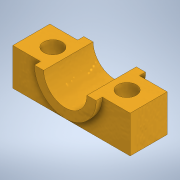
# Autodesk Inventor part: Part22
Saved by Autodesk Inventor 2020 (Build 240168000, 168)
## iProperties
Created: 2021-10-20
Part Number: Part22
Material: Brass, Soft Yellow, Welded
Document SubType Name: Modeling
Designer: simon.erikssonwestl
Density: 8.5 g/cm^3
Appearance: Weld - Brass
Author: simon.erikssonwestl
Autodesk Inventor part; units mm, degrees
ref_plane "YZ Plane" through (0, 0, 0) normal (1, 0, 0) x (0, 1, 0)
ref_plane "XZ Plane" through (0, 0, 0) normal (0, 1, 0) x (-1, 0, 0)
ref_plane "XY Plane" through (0, 0, 0) normal (0, 0, 1) x (1, 0, 0)
sketch "Sketch1" plane through (0, 0, 0) normal (0, 1, 0) x (-1, 0, 0)
  line L0 (9.5, -3) -> (-9.5, -3)
  line L1 (-9.5, -3) -> (-9.5, 3)
  line L2 (-9.5, 3) -> (9.5, 3)
  line L3 (9.5, 3) -> (9.5, -3)
  line L4 (9.5, -3) -> (-9.5, 3) construction
  line L5 (-9.5, -3) -> (9.5, 3) construction
  point P0 (0, 0)
  dimension "d0" = 19
  dimension "d1" = 6
  constraints: 12 end point, 2 midpoint, 2 parallel, 1 horizontal, 1 perpendicular
  measures "d0" distance of L1.end L2.end
  measures "d1" distance of L0.end L1.end
extrude "Extrusion1" add sketch "Sketch1" along normal blind 6
sketch "Sketch2" plane through (-9.5, 0, 3) normal (0, 0, 1) x (1, 0, 0)
  line L0 (19, 6) -> (0, 6) projected
  arc A0 (4.5, 6) -> (14.5, 6) centre (9.5, 6) ccw
  point P0 (9.5, 0)
  point P1 (14.5, 6)
  dimension "d4" = 5
  constraints: 2 point on circle, 1 centre point, 1 midpoint, 1 point on line
  measures "d4" radius of A0
extrude "Extrusion2" add sketch "Sketch2" along normal blind 1 and the other way blind 7
sketch "Sketch3" plane through (-9.5, 0, 4) normal (0, 0, 1) x (1, 0, 0)
  line L0 (14.5, 6) -> (4.5, 6) projected
  point P0 (9.5, 0)
  point P1 (9.5, 6)
  constraints: 1 midpoint
hole "Hole1" at (0, 6, 4) direction (0, 0, -1) diameter 7 end through all
sketch "Sketch4" plane through (0, 6, 0) normal (0, 1, 0) x (1, 0, 0)
  line L0 (-5, 3) -> (-9.5, 3) projected
  line L1 (9.5, 3) -> (5, 3) projected
  line L2 (-9.5, 3) -> (-9.5, -3) projected
  line L3 (9.5, -3) -> (9.5, 3) projected
  point P0 (0, 0)
  point P1 (-6, 0)
  point P2 (6, 0)
  dimension "d16" = 3
  dimension "d17" = 3
  dimension "d18" = 12
  dimension "d19" = 3.5
  dimension "d20" = 3.5
  measures "d16" distance from line of L0 point (-6, 0)
  measures "d17" distance from line of L1 point (6, 0)
  measures "d18" distance of point (-6, 0) point (6, 0)
  measures "d19" distance from line of L2 point (-6, 0)
  measures "d20" distance from line of L3 point (6, 0)
hole "Hole2" at (-6, 6, 0) at (6, 6, 0) direction (0, -1, 0) diameter 3 end through all
body "Solid1"
